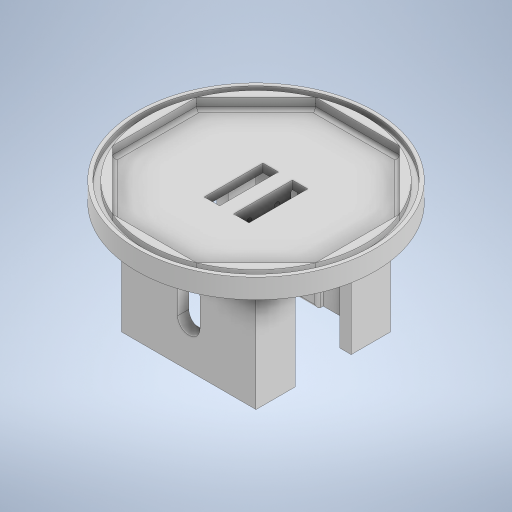
# Autodesk Inventor part: Bi_PAM
Saved by Autodesk Inventor 2024 (Build 280153000, 153)
## iProperties
Created: 2023-07-24
Part Number: Bi_PAM
Material: 일반
Document SubType Name: Modeling
Designer: jsw
Density: 1 g/cm^3
Appearance: 기본값
Author: jsw
Autodesk Inventor part; units mm, degrees
ref_plane "YZ Plane" through (0, 0, 0) normal (1, 0, 0) x (0, 1, 0)
ref_plane "XZ Plane" through (0, 0, 0) normal (0, 1, 0) x (-1, 0, 0)
ref_plane "XY Plane" through (0, 0, 0) normal (0, 0, 1) x (1, 0, 0)
sketch "스케치1" plane through (0, 0, 0) normal (0, 1, 0) x (-1, 0, 0)
  circle A0 centre (0, 0) radius 39
  circle A1 centre (0, 0) radius 42.5
  dimension "d0" = 78
  dimension "d6" = 3.5
  constraints: 2 centre point, 2 coincident
  measures "d0" diameter of A0
  measures "d6" radial gap between concentric circles of A0 A1
extrude "돌출1" add sketch "스케치1" along normal blind 7 contours A0 | A1
sketch "스케치4" plane through (0, 7, 0) normal (0, 1, 0) x (1, 0, 0)
  line L0 (15, -36.2132) -> (-15, -36.2132)
  line L1 (-15, -36.2132) -> (-36.2132, -15)
  line L2 (-36.2132, -15) -> (-36.2132, 15)
  line L3 (-36.2132, 15) -> (-15, 36.2132)
  line L4 (-15, 36.2132) -> (15, 36.2132)
  line L5 (15, 36.2132) -> (36.2132, 15)
  line L6 (36.2132, 15) -> (36.2132, -15)
  line L7 (36.2132, -15) -> (15, -36.2132)
  point P0 (0, 0)
  point P1 (0, 0)
  dimension "d17" = 30
  constraints: 16 end point, 1 coincident, 1 horizontal, 17 other
  measures "d17" distance of L0.start L0.end
extrude "돌출4" cut sketch "스케치4" against normal blind 4
fillet "모깎기1" radius 1.2 8 edges at (0, 3, -36.2132) (25.6066, 3, -25.6066) (36.2132, 3, 0) (25.6066, 3, 25.6066) (0, 3, 36.2132) (-25.6066, 3, 25.6066) (-36.2132, 3, 0) (-25.6066, 3, -25.6066)
sketch "스케치5" plane through (0, 0, 0) normal (0, -1, 0) x (1, 0, 0)
  line L0 (8, -10.5) -> (2.5, -10.5)
  line L1 (2.5, -10.5) -> (2.5, 10.5)
  line L2 (2.5, 10.5) -> (8, 10.5)
  line L3 (8, 10.5) -> (8, -10.5)
  line L4 (8, -10.5) -> (2.5, 10.5) construction
  line L5 (2.5, -10.5) -> (8, 10.5) construction
  line L6 (-2.5, -10.5) -> (-8, -10.5)
  line L7 (-8, -10.5) -> (-8, 10.5)
  line L8 (-8, 10.5) -> (-2.5, 10.5)
  line L9 (-2.5, 10.5) -> (-2.5, -10.5)
  line L10 (-2.5, -10.5) -> (-8, 10.5) construction
  line L11 (-8, -10.5) -> (-2.5, 10.5) construction
  point P0 (0, 0)
  point P1 (5.25, 0)
  point P2 (-5.25, 0)
  dimension "d21" = 5.5
  dimension "d22" = 21
  dimension "d23" = 5.5
  dimension "d24" = 21
  dimension "d25" = 5
  dimension "d27" = 2.5
  constraints: 24 end point, 4 midpoint, 4 parallel, 2 horizontal, 2 horizontal alignment, 2 perpendicular
  measures "d21" distance of L1.end L2.end
  measures "d22" distance of L0.end L1.end
  measures "d23" distance of L7.end L8.end
  measures "d24" distance of L6.end L7.end
  measures "d25" distance between parallel lines of L9 L1
  measures "d27" distance from line of L9 point (0, 0)
extrude "돌출5" cut sketch "스케치5" against normal up to surface (3 mm away)
sketch "스케치6" plane through (0, 7, 0) normal (0, 1, 0) x (1, 0, 0)
  line L0 (36.2132, -15) -> (36.2132, 15) projected
  circle A0 centre (0, 0) radius 39.1969
  circle A1 centre (0, 0) radius 41.1969
  dimension "d30" = 2
  constraints: 2 coincident, 1 centre point, 3 other
extrude "돌출6" cut sketch "스케치6" against normal blind 2
sketch "스케치7" plane through (0, 0, 0) normal (0, -1, 0) x (1, 0, 0)
  line L0 (-2.5, -10.5) -> (-2.5, 10.5) projected
  line L1 (2.5, 10.5) -> (2.5, -10.5) projected
  line L2 (-2.5, 10) -> (2.5, 10)
  line L3 (2.5, 10) -> (2.5, -10)
  line L4 (2.5, -10) -> (-2.5, -10)
  line L5 (-2.5, -10) -> (-2.5, 10)
  point P0 (0, 0)
  point P1 (0, 10)
  dimension "d33" = 20
  dimension "d34" = 10
  constraints: 8 end point, 2 parallel, 2 point on line, 1 horizontal, 1 midpoint, 1 perpendicular
  measures "d33" distance between parallel lines of L4 L2
  measures "d34" distance of point (0, 0) point (0, 10)
extrude "돌출7" add sketch "스케치7" along normal blind 6
fillet "모깎기2" radius 0.5 2 edges at (0, 0, 10) (0, 0, -10)
sketch "스케치8" plane through (2.5, 3, 10.5) normal (1, 0, 0) x (0, 0, -1)
  circle A0 centre (15.5, -5) radius 1
  line L0 (0, 0) -> (21, 0) projected
  circle A1 centre (5.5, -5) radius 1
  point P0 (10.5, -3)
  dimension "d38" = 2
  dimension "d39" = 5
  dimension "d40" = 2
  dimension "d41" = 5
  dimension "d42" = 10
  dimension "d43" = 5
  constraints: 2 centre point
  measures "d38" diameter of A0
  measures "d39" distance from line of A0.centre L0
  measures "d40" diameter of A1
  measures "d41" distance from line of L0 A1.centre
  measures "d42" distance of A1.centre A0.centre
  measures "d43" horizontal distance of A1.centre point (10.5, -3)
extrude "돌출8" cut sketch "스케치8" against normal up to surface (5 mm away)
sketch "스케치9" plane through (0, 0, 0) normal (0, -1, 0) x (1, 0, 0)
  line L0 (20, -20) -> (-20, -20)
  line L1 (-20, -20) -> (-20, 20)
  line L2 (-20, 20) -> (20, 20)
  line L3 (20, 20) -> (20, -20)
  line L4 (20, -20) -> (-20, 20) construction
  line L5 (-20, -20) -> (20, 20) construction
  line L6 (24, -24) -> (-24, -24)
  line L7 (-24, -24) -> (-24, 24)
  line L8 (-24, 24) -> (24, 24)
  line L9 (24, 24) -> (24, -24)
  line L10 (24, -24) -> (-24, 24) construction
  line L11 (-24, -24) -> (24, 24) construction
  point P0 (0, 0)
  point P1 (0, 0)
  dimension "d54" = 40
  dimension "d55" = 40
  dimension "d56" = 4
  constraints: 24 end point, 5 midpoint, 4 parallel, 2 horizontal, 2 perpendicular, 1 point on line
  measures "d54" distance of L1.end L2.end
  measures "d55" distance of L0.end L1.end
  measures "d56" distance between parallel lines of L2 L8
extrude "돌출9" add sketch "스케치9" along normal blind 40
sketch "스케치10" plane through (24, 0, 24) normal (1, 0, 0) x (0, 0, -1)
  line L0 (14, -0.5) -> (14, -6) projected
  line L1 (34, -0.5) -> (34, -6) projected
  line L2 (14, -0.5) -> (34, -0.5)
  line L3 (34, -0.5) -> (34, -40.5)
  line L4 (34, -40.5) -> (14, -40.5)
  line L5 (14, -40.5) -> (14, -0.5)
  line L6 (66.5, 0) -> (-18.5, 0) projected
  line L7 (34, -0.5) -> (34, -6) projected
  line L8 (34, -0.5) -> (14, -0.5)
  line L9 (14, -0.5) -> (14, 0)
  line L10 (14, 0) -> (34, 0)
  line L11 (34, 0) -> (34, -0.5)
  point P0 (24, 0)
  dimension "d59" = 20
  dimension "d60" = 40
  constraints: 16 end point, 4 parallel, 2 horizontal, 2 perpendicular, 1 point on line
  measures "d59" distance of L3.end L4.end
  measures "d60" distance of L2.end L3.end
extrude "돌출10" cut sketch "스케치10" against normal up to surface (4 mm away)
ref_plane "작업 평면2" through (0, 0, 24) normal (1, 0, 0) x (0, 0, -1)
mirror "미러1" about plane through (0, 0, 24) normal (1, 0, 0) of "돌출10"
sketch "스케치11" plane through (-24, 0, 24) normal (0, 0, 1) x (1, 0, 0)
  line L0 (24, -15) -> (24, -25) construction
  line L1 (20, -15) -> (20, -25)
  line L2 (28, -25) -> (28, -15)
  arc A0 (28, -15) -> (20, -15) centre (24, -15) ccw
  arc A1 (20, -25) -> (28, -25) centre (24, -25) ccw
  line L3 (0, 0) -> (48, 0) projected
  point P0 (24, 0)
  point P1 (24, -20)
  point P2 (28, -20)
  point P3 (24, 0)
  point P4 (24, -29)
  point P5 (24, -11)
  dimension "d63" = 4
  dimension "d64" = 18
  dimension "d65" = 20
  constraints: 8 end point, 6 point on circle, 4 tangent, 3 midpoint, 2 centre point, 1 parallel, 1 vertical, 1 vertical alignment
  measures "d63" distance of point (28, -20) point (24, -20)
  measures "d64" distance of point (24, -29) point (24, -11)
  measures "d65" distance from line of L3 point (24, -20)
extrude "돌출11" cut sketch "스케치11" against normal up to surface (48 mm away)
sketch "스케치12" plane through (20, 0, 20) normal (0, 0, -1) x (-1, 0, 0)
  line L0 (40, -40) -> (0, -40) projected
  line L1 (16, -40) -> (24, -40)
  line L2 (24, -40) -> (24, -30)
  line L3 (24, -30) -> (16, -30)
  line L4 (16, -30) -> (16, -40)
  line L5 (16, -15) -> (16, -25) projected
  line L6 (16, -20) -> (24, -20)
  line L7 (24, -25) -> (24, -15) projected
  line L8 (40, 0) -> (0, 0)
  line L9 (24, 0) -> (24, -10)
  line L10 (24, -10) -> (16, -10)
  line L11 (16, -10) -> (16, 0)
  point P0 (20, 0)
  point P1 (20, -40)
  point P2 (20, -40)
  dimension "d68" = 8
  dimension "d69" = 10
  dimension "d70" = 0
  constraints: 18 end point, 6 symmetric about line, 4 midpoint, 2 parallel, 2 point on line, 1 horizontal, 1 perpendicular
  measures "d68" distance of L3.end L2.end
  measures "d69" distance of L1.end L2.end
  measures "d70" distance of point (20, -40) point (20, -40)
extrude "돌출12" add sketch "스케치12" along normal blind 2
fillet "모깎기3" radius 1 7 edges at (-4, -35, 18) (4, -35, 18) (-4, -5, 18) (4, -5, 18) (0, -10, 18) (0, -30, 18) (0, -40, 18)
ref_plane "작업 평면3" through (24, 0, 0) normal (0, 0, -1) x (-1, 0, 0)
mirror "미러2" about plane through (24, 0, 0) normal (0, 0, -1) of "모깎기3", "돌출12"
equation "\"d27\" = 0.5 * d25"
